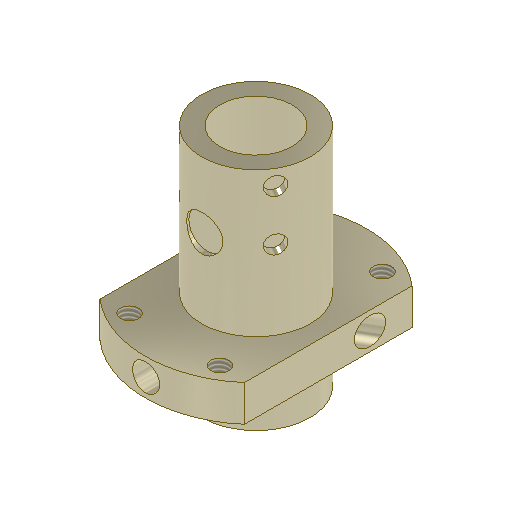
# Autodesk Inventor part: collimator
Saved by Autodesk Inventor 2022.4 (Build 264492000, 492)
## iProperties
Category: -
Company: Universiteit van Amsterdam
Created: 2023-08-21
Part Number: collimator
Material: Nickel-Copper Alloy 400
Document SubType Name: Modeling
Designer: RbSrWorkstation1
Density: 8.83 g/cm^3
Appearance: Nickel
User Status: Work in Progress
Author: RbSrWorkstation1
Revision Number: A
Autodesk Inventor part; units mm, degrees
ref_plane "YZ Plane" through (0, 0, 0) normal (1, 0, 0) x (0, 1, 0)
sketch "Sketch1" plane through (0, 0, 0) normal (0, 1, 0) x (-1, 0, 0)
  circle A0 centre (0, 0) radius 6
  circle A1 centre (0, 0) radius 4
  circle A2 centre (0, 0) radius 12.25
  line L0 (-8, 9.277) -> (-8, -9.277)
  line L1 (8, -9.277) -> (8, 9.277)
  dimension "d0" = 12
  dimension "d59" = 16
  dimension "d60" = 24.5
  dimension "d61" = 8
  constraints: 4 end point, 4 point on circle, 3 centre point, 3 coincident, 2 parallel, 1 vertical
  measures "d0" diameter of A0
  measures "d59" distance between parallel lines of L1 L0
  measures "d60" diameter of A2
  measures "d61" diameter of A1
extrude "Extrusion13" add sketch "Sketch1" along normal blind 16 contours A0
extrude "Extrusion14" add sketch "Sketch1" against normal blind 4 contours A0 | L1 A2 L0
sketch "Sketch9" plane through (0, -4, 0) normal (0, -1, 0) x (1, 0, 0)
  circle A0 centre (0, 0) radius 6
  circle A1 centre (0, 0) radius 4.5
  dimension "d64" = 12
  dimension "d65" = 9
  constraints: 2 centre point, 2 coincident
  measures "d64" diameter of A0
  measures "d65" diameter of A1
extrude "Extrusion15" add sketch "Sketch9" along normal blind 5
sketch "Sketch10" plane through (0, -4, 0) normal (0, -1, 0) x (1, 0, 0)
  line L0 (-5, 9) -> (5, -9) construction
  point P0 (0, 0)
  point P1 (5, 9)
  point P2 (-5, -9)
  point P3 (0, 0)
  dimension "d75" = 10
  dimension "d76" = 18
  constraints: 2 end point, 2 horizontal alignment, 2 vertical alignment, 1 coincident, 1 midpoint
  measures "d75" distance of point (5, 9) L0.start
  measures "d76" distance of point (-5, -9) L0.start
hole "Hole1" at (-5, -4, 9) at (5, -4, 9) at (-5, -4, -9) at (5, -4, -9) direction (0, 1, 0) diameter 2.013 end through all thread size "M2.5x0.45" class "6H" standard "ISO Metric profile"
ref_plane "Work Plane6" through (0, 8.7, 0) normal (0, 1, 0) x (-1, 0, 0)
sketch "Sketch11" plane through (0, 8.7, 0) normal (0, 1, 0) x (-1, 0, 0)
  line L0 (0, 10.4415) -> (2, 10.4415)
  line L1 (2, 10.4415) -> (2, 5.4415)
  line L2 (2, 5.4415) -> (0, 5.4415)
  line L3 (0, 5.4415) -> (0, 10.4415)
  line L4 (4.3301, 2.5) -> (4.8301, 1.634)
  line L5 (4.8301, 1.634) -> (9.1603, 4.134)
  line L6 (9.1603, 4.134) -> (8.6603, 5)
  line L7 (8.6603, 5) -> (4.3301, 2.5)
  line L8 (-4.3301, 2.5) -> (-3.8301, 3.366)
  line L9 (-3.8301, 3.366) -> (-8.1603, 5.866)
  line L10 (-8.1603, 5.866) -> (-8.6603, 5)
  line L11 (-8.6603, 5) -> (-4.3301, 2.5)
  point P0 (0, 0)
  dimension "d78" = 120
  dimension "d79" = 60
  dimension "d80" = 5
  dimension "d81" = 5
  dimension "d82" = 5.4415
  dimension "d83" = 4
  dimension "d84" = 2
  dimension "d85" = 2
  dimension "d86" = 5
  constraints: 24 end point, 6 parallel, 3 perpendicular, 3 point on line, 2 equal length, 1 horizontal
  measures "d78" angle of L9 L7
  measures "d79" angle of L9 L3
  measures "d80" distance from line of point (0, 0) L8
  measures "d81" distance from line of L4 point (0, 0)
  measures "d82" distance from line of L2 point (0, 0)
  measures "d83" diameter of L1 L3
  measures "d84" diameter of L5 L7
  measures "d85" diameter of L9 L11
  measures "d86" distance of L0.end L1.end
revolve "Revolution1" cut sketch "Sketch11" angle 360 about axis through (8.6603, 8.7, 5) along (-0.8660254, 0, -0.5) contours L11 L10 L9 L8
revolve "Revolution2" cut sketch "Sketch11" angle 360 about axis through (0, 8.7, 5.4415) along (0, 0, 1) contours L0 L1 L2 L3
revolve "Revolution3" cut sketch "Sketch11" angle 360 about axis through (-8.6603, 8.7, 5) along (0.8660254, 0, -0.5) contours L7 L6 L5 L4
ref_plane "Work Plane7" through (0, 14.3, 0) normal (0, 1, 0) x (-1, 0, 0)
sketch "Sketch12" plane through (0, 14.3, 0) normal (0, 1, 0) x (-1, 0, 0)
  line L0 (-3.8301, 3.366) -> (-8.1603, 5.866) projected
  line L1 (-8.1603, 5.866) -> (-8.6603, 5) projected
  line L2 (-8.6603, 5) -> (-4.3301, 2.5) projected
  line L3 (-4.3301, 2.5) -> (-3.8301, 3.366) projected
  point P0 (0, 0)
revolve "Revolution4" cut sketch "Sketch12" angle 360 about axis through (8.6603, 14.3, 5) along (-0.8660254, 0, -0.5)
pattern_circular "Circular Pattern3" count 3 over 360 about axis through (0, -10, 0) along (0, 1, 0) of "Revolution4"
ref_plane "Work Plane9" through (0, -2, 0) normal (0, 1, 0) x (-1, 0, 0)
sketch "Sketch13" plane through (0, -2, 0) normal (0, 1, 0) x (-1, 0, 0)
  line L0 (0, 20) -> (0, 0)
  line L1 (0, 0) -> (1.5, 0)
  line L2 (1.5, 0) -> (1.5, 20)
  line L3 (1.5, 20) -> (0, 20)
  dimension "d106" = 3
  dimension "d107" = 20
  constraints: 8 end point, 3 perpendicular, 1 vertical
  measures "d106" diameter of L2 L0
  measures "d107" distance of L1.end L2.end
revolve "Revolution5" cut sketch "Sketch13" angle 360 about axis through (0, -2, 20) along (0, 0, -1)
pattern_circular "Circular Pattern4" count 3 over 360 about axis through (0, -10, 0) along (0, 1, 0) of "Revolution5"
body "Solid2"
